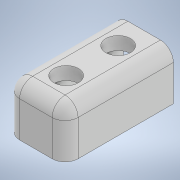
# Autodesk Inventor part: Full
Saved by Autodesk Inventor 2021 (Build 250183000, 183)
## iProperties
Created: 2020-05-12
Part Number: Full
Material: Generic
Document SubType Name: Modeling
Designer: andre
Density: 1 g/cm^3
Appearance: Default
Author: andre
## iProperties of the stored document _3DPrint.ipt
Created: 2020-05-21
Part Number: _3DPrint
Material: Generic
Document SubType Name: Modeling
Designer: andre
Density: 1 g/cm^3
Appearance: Default
Author: andre
Autodesk Inventor part; units mm, degrees
ref_plane "YZ Plane" through (0, 0, 0) normal (1, 0, 0) x (0, 1, 0)
ref_plane "XZ Plane" through (0, 0, 0) normal (0, 1, 0) x (-1, 0, 0)
ref_plane "XY Plane" through (0, 0, 0) normal (0, 0, 1) x (1, 0, 0)
sketch "Base" plane through (0, 0, 0) normal (0, 1, 0) x (-1, 0, 0)
  line L0 (0, 25) -> (0, -175)
  line L1 (0, -175) -> (54, -175)
  line L2 (54, -175) -> (54, 25)
  line L3 (54, 25) -> (0, 25)
  dimension "d6" = 200
  dimension "d7" = 54
  constraints: 8 end point, 2 perpendicular, 1 vertical
  measures "d6" distance between parallel lines of L1 L3
  measures "d7" distance of L0.end L1.end
extrude "Extrusion2" add sketch "Base" along normal blind 45
sketch "Top" plane through (0, 45, 0) normal (0, 1, 0) x (1, 0, 0)
  circle A0 centre (-27, 51) radius 14.25
  circle A1 centre (-27, 3) radius 14.25
  circle A2 centre (-27, 99) radius 14.25
  circle A3 centre (-27, 147) radius 14.25
  line L0 (0, 175) -> (-54, 175) projected
  line L1 (-54, 175) -> (-54, -25) projected
  line L2 (-54, -25) -> (0, -25) construction
  line L3 (-27, -25) -> (-27, 175) construction
  circle A4 centre (-27, 3) radius 11.4
  circle A5 centre (-27, 51) radius 11.4
  circle A6 centre (-27, 99) radius 11.4
  circle A7 centre (-27, 147) radius 11.4
  point P0 (-27, 75)
  dimension "d10" = 28.5
  dimension "d11" = 28.5
  dimension "d12" = 28.5
  dimension "d13" = 28.5
  dimension "d14" = 48
  dimension "d15" = 48
  dimension "d16" = 48
  dimension "d27" = 22.8
  dimension "d28" = 22.8
  dimension "d29" = 22.8
  dimension "d30" = 22.8
  dimension "d31" = 24
  dimension "d32" = 100
  dimension "d35" = 28
  constraints: 8 centre point, 4 coincident, 3 midpoint, 3 vertical alignment, 2 end point, 1 point on line
  measures "d10" diameter of A0
  measures "d11" diameter of A1
  measures "d12" diameter of A2
  measures "d13" diameter of A3
  measures "d14" distance of A0.centre A1.centre
  measures "d15" distance of A2.centre A0.centre
  measures "d16" distance of A3.centre A2.centre
  measures "d27" diameter of A4
  measures "d28" diameter of A5
  measures "d29" diameter of A6
  measures "d30" diameter of A7
  measures "d31" distance of point (-27, 75) A2.centre
  measures "d32" distance from line of point (-27, 75) L0
  measures "d35" distance from line of A1.centre L2
extrude "Extrusion3" cut sketch "Top" against normal up to next contours A4 | A5 | A6 | A7
sketch "Walls" plane through (0, 0, 0) normal (0, -1, 0) x (1, 0, 0)
  line L0 (-8, 17) -> (-46, 17)
  line L1 (-46, 17) -> (-46, -167)
  line L2 (-46, -167) -> (-8, -167)
  line L3 (-8, -167) -> (-8, 17)
  line L4 (-54, 25) -> (0, 25) projected
  line L5 (0, -175) -> (-54, -175) projected
  line L6 (0, 25) -> (0, -175) projected
  line L7 (-54, -175) -> (-54, 25) projected
  point P0 (0, 0)
  dimension "d21" = 8
  dimension "d22" = 8
  dimension "d23" = 8
  dimension "d24" = 8
  dimension "d33" = 38
  constraints: 8 end point, 2 parallel, 1 horizontal, 1 perpendicular
  measures "d21" distance between parallel lines of L4 L0
  measures "d22" distance between parallel lines of L5 L2
  measures "d23" distance between parallel lines of L6 L3
  measures "d24" distance between parallel lines of L7 L1
  measures "d33" distance between parallel lines of L1 L3
extrude "Extrusion4" cut sketch "Walls" against normal blind 33 contours L3 L2 L1 L0
fillet "Fillet1" radius 12 8 edges at (-27, 45, 25) (-54, 45, -75) (0, 45, -75) (0, 22.5, 25) (-54, 22.5, 25) (0, 22.5, -175) (-27, 45, -175) (-54, 22.5, -175)
sketch "Sketch7" plane through (-54, 0, -163) normal (-1, 0, 0) x (0, 0, 1)
  line L0 (0, 33) -> (176, 33) projected
  line L1 (0, 0) -> (176, 0) projected
  circle A0 centre (88, 0) radius 3
  point P0 (163, 0)
  dimension "d40" = 6
  constraints: 1 centre point, 1 midpoint
  measures "d40" diameter of A0
extrude "Extrusion5" cut sketch "Sketch7" against normal up to surface (8 mm away)
fillet "Fillet2" radius 5 4 edges at (-8, 16.5, 17) (-46, 16.5, 17) (-8, 16.5, -167) (-46, 16.5, -167)
sketch "Sketch10" plane through (-12, 0, -175) normal (0, 0, -1) x (-1, 0, 0)
  line L0 (83.179, 90.3723) -> (-24.5359, 90.3723)
  line L1 (-24.5359, 90.3723) -> (-24.5359, -32.2986)
  line L2 (-24.5359, -32.2986) -> (83.179, -32.2986)
  line L3 (83.179, -32.2986) -> (83.179, 90.3723)
  point P0 (-12, 0)
  constraints: 8 end point, 2 parallel, 1 horizontal, 1 perpendicular
extrude "Half" cut sketch "Sketch10" against normal blind 100
sketch "Sketch13" plane through (0, 0, 0) normal (0, -1, 0) x (1, 0, 0)
  line L0 (-8, 12) -> (-8, -75) projected
  line L1 (-8, -51) -> (-4, -51)
  line L2 (-4, -51) -> (-4, -43)
  line L3 (-4, -43) -> (-8, -43)
  line L4 (-8, -43) -> (-8, -51)
  circle A0 centre (-27, -51) radius 11.4 construction
  line L5 (0, 13) -> (0, -75) construction
  line L6 (0, -35) -> (-53.8786, -35) construction
  circle A1 centre (-27, -3) radius 11.4 construction
  line L7 (-8, -82) -> (-8, 5)
  line L8 (-8, -19) -> (-4, -19)
  line L9 (-4, -19) -> (-4, -27)
  line L10 (-4, -27) -> (-8, -27)
  line L11 (-8, -27) -> (-8, -19)
  line L12 (-27, -51) -> (-27, -3) construction
  line L13 (-46, -51) -> (-50, -51)
  line L14 (-50, -51) -> (-50, -43)
  line L15 (-50, -43) -> (-46, -43)
  line L16 (-46, -43) -> (-46, -51)
  line L17 (-46, -19) -> (-50, -19)
  line L18 (-46, -27) -> (-46, -19)
  line L19 (-50, -19) -> (-50, -27)
  line L20 (-50, -27) -> (-46, -27)
  point P0 (0, 0)
  point P1 (-8, -19)
  point P2 (-8, -27)
  point P3 (-8, -43)
  dimension "d50" = 4
  dimension "d52" = 8
  dimension "d53" = 0
  dimension "d54" = 8
  constraints: 38 end point, 14 symmetric about line, 3 point on line, 2 coincident, 2 horizontal, 2 parallel, 1 perpendicular, 1 vertical
  measures "d50" distance between parallel lines of L0 L2
  measures "d52" distance of L1.end L2.end
  measures "d53" distance from line of L12.start L1
  measures "d54" distance between parallel lines of L6 L3
extrude "Extrusion7" cut sketch "Sketch13" against normal blind 5
equation "\"d11\" = d10"
equation "\"d12\" = d10"
equation "\"d13\" = d10"
equation "\"d15\" = d14"
equation "\"d16\" = d14"
equation "\"d28\" = d27"
equation "\"d29\" = d27"
equation "\"d30\" = d27"
equation "\"d31\" = 0.5 * d14"
equation "\"d32\" = 0.5 * d6"
equation "\"d22\" = d21"
equation "\"d23\" = d21"
equation "\"d24\" = d23"
body "Solid2"
